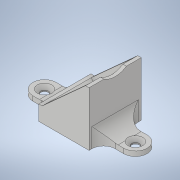
# Autodesk Inventor part: Kamerahalterung_Winkel_45
Saved by Autodesk Inventor 2021 (Build 250183000, 183)
## iProperties
Created: 2020-05-20
Part Number: Kamerahalterung_Winkel_45
Material: Generisch
Document SubType Name: Modeling
Designer: 111162002
Density: 1 g/cm^3
Appearance: Vorgabe
Author: 111162002
Autodesk Inventor part; units mm, degrees
ref_plane "YZ Plane" through (0, 0, 0) normal (1, 0, 0) x (0, 1, 0)
ref_plane "XZ Plane" through (0, 0, 0) normal (0, 1, 0) x (-1, 0, 0)
ref_plane "XY Plane" through (0, 0, 0) normal (0, 0, 1) x (1, 0, 0)
sketch "Skizze1" plane through (0, 0, 0) normal (0, 0, 1) x (1, 0, 0)
  line L0 (0, 0) -> (0, 10)
  line L1 (0, 10) -> (33.8, 43.8)
  line L2 (33.8, 43.8) -> (33.8, 0)
  line L3 (33.8, 0) -> (0, 0)
  line L4 (0, 10) -> (-3.5753, 13)
  line L5 (-3.5753, 13) -> (-6.5753, 13)
  line L6 (-6.5753, 13) -> (-6.5753, 0)
  line L7 (-6.5753, 0) -> (0, 0)
  line L8 (33.8, 43.8) -> (33.8, 46.8)
  line L9 (33.8, 46.8) -> (36.8, 46.8)
  line L10 (36.8, 46.8) -> (36.8, 0)
  line L11 (33.8, 0) -> (36.8, 0)
  dimension "d0" = 135
  dimension "d1" = 95
  dimension "d6" = 33.8
  dimension "d8" = 3
  dimension "d9" = 10
  dimension "d11" = 3
  dimension "d13" = 3
  dimension "d14" = 3
  constraints: 24 end point, 4 parallel, 3 perpendicular, 1 collinear, 1 horizontal, 1 point on line, 1 vertical
  measures "d0" angle of L1 L0
  measures "d1" angle of L1 L4
  measures "d6" horizontal distance of L0.end L1.end
  measures "d8" distance from line of L5 L0.end
  measures "d9" distance from line of L3 L0.end
  measures "d11" distance from line of L9 L1.end
  measures "d13" distance of L4.end L5.end
  measures "d14" distance of L8.end L9.end
extrude "Extrusion1" add sketch "Skizze1" along normal blind 45
sketch "Skizze3" plane through (0, 0, 0) normal (0, 0, -1) x (-1, 0, 0)
  line L0 (-33.8, 46.8) -> (3.5753, 13)
  line L1 (-33.8, 43.8) -> (0, 10) projected
  line L2 (3.5753, 13) -> (0, 10)
  line L3 (0, 10) -> (-33.8, 43.8)
  line L4 (-33.8, 46.8) -> (-33.8, 43.8) projected
  line L5 (-33.8, 43.8) -> (-33.8, 46.8)
  constraints: 8 end point, 2 collinear
sketch "Skizze4" plane through (0, 0, 45) normal (0, 0, 1) x (1, 0, 0)
  line L0 (0, 10) -> (-3.5753, 13) projected
  line L1 (33.8, 43.8) -> (0, 10) projected
  line L2 (0, 10) -> (33.8, 43.8)
  line L3 (33.8, 46.8) -> (33.8, 43.8) projected
  line L4 (33.8, 43.8) -> (33.8, 46.8)
  line L5 (33.8, 46.8) -> (-3.5753, 13)
  line L6 (-3.5753, 13) -> (0, 10)
  point P0 (0, 0)
  constraints: 8 end point, 2 collinear
extrude "Extrusion3" add sketch "Skizze4" against normal blind 3
extrude "Extrusion4" add sketch "Skizze3" against normal blind 3
sketch "Skizze5" plane through (-6.5753, 0, 0) normal (0, -1, 0) x (1, 0, 0)
  line L0 (0, 45) -> (43.3753, 45) projected
  line L1 (0, 0) -> (43.3753, 0) projected
  line L2 (0, 0) -> (0, 45) projected
  line L3 (0, 12.5) -> (-27.5, 12.5)
  line L4 (-27.5, 12.5) -> (-27.5, 32.5)
  line L5 (-27.5, 32.5) -> (0, 32.5)
  line L6 (0, 32.5) -> (0, 12.5)
  circle A0 centre (-17.5, 22.5) radius 3.25
  line L7 (43.3753, 0) -> (43.3753, 45) projected
  line L8 (43.3753, 32.5) -> (70.8753, 32.5)
  line L9 (70.8753, 32.5) -> (70.8753, 12.5)
  line L10 (70.8753, 12.5) -> (43.3753, 12.5)
  line L11 (43.3753, 12.5) -> (43.3753, 32.5)
  circle A1 centre (60.8753, 22.5) radius 3.25
  point P0 (6.5753, 0)
  dimension "d71" = 6.5
  dimension "d72" = 10
  dimension "d73" = 20
  dimension "d74" = 10
  dimension "d75" = 27.5
  dimension "d76" = 6.5
  dimension "d77" = 27.5
  dimension "d78" = 20
  dimension "d79" = 10
  dimension "d80" = 10
  dimension "d81" = 12.5
  dimension "d82" = 12.5
  constraints: 16 end point, 4 parallel, 2 centre point, 2 horizontal, 2 perpendicular, 2 point on line
  measures "d71" diameter of A1
  measures "d72" distance from line of L9 A1.centre
  measures "d73" distance of L8.end L9.end
  measures "d74" distance from line of L10 A1.centre
  measures "d75" distance of L8.start L8.end
  measures "d76" diameter of A0
  measures "d77" distance of L4.end L5.end
  measures "d78" distance of L3.end L4.end
  measures "d79" distance from line of L3 A0.centre
  measures "d80" distance from line of L4 A0.centre
  measures "d81" distance between parallel lines of L0 L8
  measures "d82" distance between parallel lines of L0 L5
extrude "Extrusion5" add sketch "Skizze5" against normal blind 4.1 contours L2 L3 L4 L5 | L8 L9 L10 L7
sketch "Skizze6" plane through (0, 10, 42) normal (-0.7071068, 0.7071068, 0) x (0.7071068, 0.7071068, 0)
  line L0 (12.4, 24.1) -> (2.6, 24.1)
  line L1 (2.6, 24.1) -> (2.6, 14.9)
  line L2 (2.6, 14.9) -> (12.4, 14.9)
  line L3 (12.4, 14.9) -> (12.4, 24.1)
  circle A0 centre (7.5, 19.5) radius 3.25
  line L4 (47.8004, 39) -> (0, 39) projected
  line L5 (0, 39) -> (0, 0) projected
  point P0 (-7.0711, 42)
  point P1 (0, -3)
  dimension "d40" = 9.8
  dimension "d41" = 9.2
  dimension "d42" = 6.5
  dimension "d43" = 4.9
  dimension "d44" = 4.6
  dimension "d45" = 19.5
  dimension "d46" = 7.5
  constraints: 8 end point, 2 parallel, 1 centre point, 1 horizontal, 1 perpendicular
  measures "d40" distance of L1.end L2.end
  measures "d41" distance of L2.end L0.start
  measures "d42" diameter of A0
  measures "d43" distance from line of L3 A0.centre
  measures "d44" distance from line of L0 A0.centre
  measures "d45" distance from line of L4 A0.centre
  measures "d46" distance from line of L5 A0.centre
extrude "Extrusion6" cut sketch "Skizze6" against normal blind 1.5
extrude "Extrusion7" cut sketch "Skizze6" against normal up to surface contours A0 surface through (-6.5753, 0, 0) normal (0, -1, 0)
chamfer "Fase1" distance 3 angle 45 2 edges at (-27.3253, 4.1, 22.5) (51.05, 4.1, 22.5)
sketch "Skizze7" plane through (33.8, 43.8, 42) normal (-1, 0, 0) x (0, 0, 1)
  circle A0 centre (-19.5, 17.25) radius 17.2
  line L0 (-39, 0) -> (0, 0) projected
  line L1 (0, -33.8) -> (0, 0) projected
  point P0 (-42, -43.8)
  point P1 (3, 0)
  point P2 (0, -24.9676)
  dimension "d57" = 34.4
  dimension "d58" = 17.25
  dimension "d59" = 19.5
  constraints: 1 centre point
  measures "d57" diameter of A0
  measures "d58" distance from line of L0 A0.centre
  measures "d59" distance from line of L1 A0.centre
extrude "Extrusion8" cut sketch "Skizze7" against normal up to surface (3 mm away)
fillet "Rundung1" [suppressed]
fillet "Rundung2" radius 10 8 edges at (-6.5753, 2.05, 32.5) (36.8, 2.05, 32.5) (36.8, 2.05, 12.5) (-6.5753, 2.05, 12.5) (-34.0753, 2.05, 32.5) (-34.0753, 2.05, 12.5) (64.3, 2.05, 32.5) (64.3, 2.05, 12.5)
fillet "Rundung4" radius 12.5 6 edges at (-6.5753, 4.1, 7.5001) (-6.5753, 4.1, 22.5) (-6.5753, 4.1, 37.5) (36.8, 4.1, 37.4999) (36.8, 4.1, 22.5) (36.8, 4.1, 7.5001)
ref_plane "Arbeitsebene1" through (6.7175, 3.2825, 42) normal (-0.7071068, 0.7071068, 0) x (0, 0, -1)
sketch "Skizze12" plane through (6.7175, 3.2825, 42) normal (-0.7071068, 0.7071068, 0) x (0, 0, -1)
  circle A0 centre (19.5, -7.5) radius 6.25
  line L0 (24.1, -12.4) -> (14.9, -12.4) projected
  line L1 (14.9, -12.4) -> (14.9, -2.6) projected
  circle A1 centre (19.5, -7.5) radius 3.25 projected
  line L2 (24.1, -2.6) -> (24.1, -12.4) projected
  line L3 (14.9, -2.6) -> (24.1, -2.6) projected
  line L4 (14.9, -12.4) -> (14.9, -2.6) projected
  line L5 (24.1, -12.4) -> (14.9, -12.4) projected
  line L6 (42, -42.5431) -> (-3, -42.5431) projected
  line L7 (-3, -42.5431) -> (-3, 4.6421) projected
  line L8 (-3, 4.6421) -> (42, 4.6421) projected
  line L9 (42, 4.6421) -> (42, -42.5431) projected
  circle A2 centre (19.5, -7.5) radius 3.25 projected
  line L10 (42, -42.5431) -> (-3, -42.5431) projected
  line L11 (-3, -42.5431) -> (-3, 4.6421) projected
  line L12 (-3, 4.6421) -> (42, 4.6421) projected
  line L13 (42, 4.6421) -> (42, -42.5431) projected
  circle A3 centre (19.5, -7.5) radius 3.25 projected
  line L14 (42, -42.5431) -> (-3, -42.5431) projected
  line L15 (-3, -42.5431) -> (-3, 4.6421) projected
  line L16 (-3, 4.6421) -> (42, 4.6421) projected
  line L17 (42, 4.6421) -> (42, -42.5431) projected
  circle A4 centre (19.5, -7.5) radius 3.25 projected
  point P0 (42, 7.0711)
  point P1 (14.9, -3.2689)
  point P2 (14.9, -11.7311)
  dimension "d98" = 12.5
  dimension "d99" = 4.9
  dimension "d100" = 4.6
  constraints: 1 centre point
  measures "d98" diameter of A0
  measures "d99" distance from line of A0.centre L0
  measures "d100" distance from line of L1 A0.centre
extrude "Extrusion10" cut sketch "Skizze12" against normal blind 18.5 contours A0 L2 | L2 A0 L0 L1 L3 | L3 A0 | A0 L0 | L1 A0 | A1
chamfer "Fase4" distance 3 angle 45 1 edges at (9.7213, 6.2891, 22.5)
equation "\"d43\" = 0.5 * d40"
equation "\"d44\" = 0.5 * d41"
equation "\"d59\" = d45"
